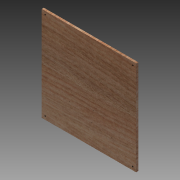
# Autodesk Inventor part: Print_TopPlate
Saved by Autodesk Inventor 2014 (Build 180170000, 170)
## iProperties
Created: 2013-12-17
Part Number: Print_TopPlate
Material: Birch
Document SubType Name: Modeling
Designer: Bram
Density: 0.512 g/cm^3
Appearance: Birch - Natural Medium Gloss
Author: Bram
Autodesk Inventor part; units mm, degrees
ref_plane "YZ Plane" through (0, 0, 0) normal (1, 0, 0) x (0, 1, 0)
ref_plane "XZ Plane" through (0, 0, 0) normal (0, 1, 0) x (-1, 0, 0)
ref_plane "XY Plane" through (0, 0, 0) normal (0, 0, 1) x (1, 0, 0)
sketch "Sketch1" plane through (0, 0, 0) normal (0, 1, 0) x (-1, 0, 0)
  line L0 (0, 0) -> (225, 0)
  line L1 (225, 0) -> (225, 225)
  line L2 (225, 225) -> (0, 225)
  line L3 (0, 225) -> (0, 0)
  dimension "d0" = 225
  dimension "d1" = 225
  constraints: 8 end point, 2 parallel, 1 horizontal, 1 perpendicular
  measures "d0" distance of L2.end L1.end
  measures "d1" distance of L1.end L0.end
extrude "Extrusion1" add sketch "Sketch1" along normal blind 5
sketch "Sketch2" plane through (0, 5, 0) normal (0, 1, 0) x (1, 0, 0)
  line L0 (-217, -8) -> (-8, -8)
  line L1 (-8, -8) -> (-8, -217)
  line L2 (-8, -217) -> (-217, -217)
  line L3 (-217, -217) -> (-217, -8)
  circle A0 centre (-217, -8) radius 1.5
  circle A1 centre (-8, -8) radius 1.5
  circle A2 centre (-217, -217) radius 1.5
  circle A3 centre (-8, -217) radius 1.5
  dimension "d4" = 209
  dimension "d5" = 209
  dimension "d6" = 3
  dimension "d7" = 3
  dimension "d8" = 3
  dimension "d9" = 3
  constraints: 8 end point, 4 centre point, 4 coincident, 2 parallel, 1 horizontal, 1 perpendicular
  measures "d4" distance of L1.end L2.end
  measures "d5" distance of L0.end L1.end
  measures "d6" diameter of A0
  measures "d7" diameter of A1
  measures "d8" diameter of A2
  measures "d9" diameter of A3
extrude "Extrusion2" cut sketch "Sketch2" against normal blind 5 contours L3 A0 L0 | L0 A0 L3 | A1 L1 L0 | L0 L1 A1 | A2 L2 L3 | L3 L2 A2 | A3 L2 L1 | L1 L2 A3
body "Solid1"
